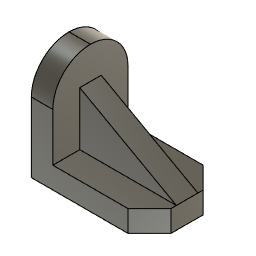
A1 (Autodesk Fusion 360 design; units mm, degrees)
Autodesk Fusion 360 part; units mm, degrees
note: some values were not read from the file. Set by a fixed rule: which sketch regions a step uses.
sketch "Sketch1" plane through (0, 0, 0) normal (0, 0, 1) x (1, 0, 0)
  line L0 (-20.0087, 11.2989) -> (639.9913, 11.2989)
  line L1 (639.9913, 11.2989) -> (639.9913, -408.7011)
  line L2 (639.9913, -408.7011) -> (-20.0087, -408.7011)
  line L3 (-20.0087, -408.7011) -> (-20.0087, 11.2989)
  line L4 (519.9913, -288.7011) -> (639.9913, -288.7011)
  line L5 (639.9913, -288.7011) -> (639.9913, -408.7011)
  line L6 (639.9913, -408.7011) -> (519.9913, -408.7011)
  line L7 (519.9913, -408.7011) -> (519.9913, -288.7011)
  line L8 (519.9913, 11.2989) -> (639.9913, 11.2989)
  line L9 (639.9913, 11.2989) -> (639.9913, -108.7011)
  line L10 (639.9913, -108.7011) -> (519.9913, -108.7011)
  line L11 (519.9913, -108.7011) -> (519.9913, 11.2989)
  line L12 (519.9913, -408.7011) -> (639.9913, -288.7011)
  line L13 (519.9913, 11.2989) -> (639.9913, -108.7011)
  dimension "d1" = 660
  dimension "d2" = 420
  dimension "d3" = 120
  dimension "d4" = 120
  dimension "d5" = 120
  dimension "d6" = 120
  constraint horizontal L0
  constraint vertical L1
  constraint horizontal L2
  constraint vertical L3
  constraint horizontal L4
  constraint vertical L5
  constraint horizontal L6
  constraint vertical L7
  constraint collinear L2 L6
  constraint collinear L1 L5
  constraint horizontal L8
  constraint vertical L9
  constraint horizontal L10
  constraint vertical L11
  constraint coincident L0 L8.start
  constraint collinear L1 L9
  measures "d1" distance of L0.start L0.end
  measures "d2" distance of L0.start L2.end
  measures "d3" distance of L4.start L4.end
  measures "d4" distance of L4.start L6.end
  measures "d5" distance of L8.start L0.end
  measures "d6" distance of L8.start L10.end
extrude "Extrude2" add sketch "Sketch1" along normal blind 120 contours L0 L1 L2 L3 L4 L7 L10 L11 | L10 L11 L13 | L4 L7 L12 makes body 1
sketch "Sketch2" plane through (0, 0, 120) normal (0, 0, 1) x (-1, 0, 0)
  line L0 (-519.9913, 408.7011) -> (-639.9913, 288.7011)
  line L1 (-639.9913, 288.7011) -> (-639.9913, 108.7011)
  line L2 (-639.9913, 108.7011) -> (-519.9913, -11.2989)
  line L3 (-519.9913, -11.2989) -> (20.0087, -11.2989)
  line L4 (20.0087, -11.2989) -> (20.0087, 408.7011)
  line L5 (20.0087, 408.7011) -> (-519.9913, 408.7011)
  line L6 (20.0087, -11.2989) -> (-99.9913, -11.2989)
  line L7 (-99.9913, -11.2989) -> (-99.9913, 408.7011)
  line L8 (-99.9913, 408.7011) -> (20.0087, 408.7011)
  line L9 (20.0087, 408.7011) -> (20.0087, -11.2989)
  dimension "d11" = 120
  constraint horizontal L6
  constraint vertical L7
  constraint horizontal L8
  constraint vertical L9
  constraint coincident L3.end L4.start
  measures "d11" distance of L3.end L6.end
extrude "Extrude3" add sketch "Sketch2" along normal blind 270 contours L3 L4 L5 L6 L7 L8 L9 bodies 1
sketch "Sketch3" plane through (0, -408.7011, 0) normal (0, -1, 0) x (1, 0, 0)
  line L0 (-20.0087, 0) -> (519.9913, 0)
  line L1 (519.9913, 0) -> (519.9913, 120)
  line L2 (519.9913, 120) -> (99.9913, 120)
  line L3 (99.9913, 120) -> (99.9913, 390)
  line L4 (99.9913, 390) -> (-20.0087, 390)
  line L5 (-20.0087, 390) -> (-20.0087, 0)
  line L6 (99.9913, 120) -> (99.9913, 420)
  line L7 (99.9913, 120) -> (639.9913, 120)
  line L8 (99.9913, 420) -> (639.9913, 120)
  dimension "d14" = 300
  dimension "d15" = 540
  constraint coincident L2.end L3.start
  constraint perpendicular L4 L6
  constraint perpendicular L1 L7
  measures "d14" distance of L2.end L6.end
  measures "d15" distance of L2.end L7.end
extrude "Extrude4" add sketch "Sketch3" along normal blind 120 separate body contours L2 L3 L6 L7 L8 makes body 2
move_body "Move1" bodies 2 to x (1, 0, 0) y (0, 1, 0) z (0, 0, 1) at (-487.7424, -224.6451, -38.3321)
move_body "Move2" bodies 2 to x (1, 0, 0) y (0, 1, 0) z (0, 0, 1) at (490, 500, 40)
move_body "Move3" bodies 2 to x (1, 0, 0) y (0, 1, 0) z (0, 0, 1) at (0, -5, 0)
sketch "Sketch5" plane through (-20.0087, 0, 0) normal (-1, 0, 0) x (0, -1, 0)
  line L0 (-11.2989, 0) -> (408.7011, 0)
  line L1 (408.7011, 0) -> (408.7011, 390)
  line L2 (408.7011, 390) -> (-11.2989, 390)
  line L3 (-11.2989, 390) -> (-11.2989, 0)
  line L4 (-11.2989, 390) -> (408.7011, 390)
  line L5 (408.7011, 390) -> (408.7011, 390.0002)
  line L6 (198.6557, 600.0002) -> (198.7011, 600.0002)
  line L7 (-11.2988, 390.0783) -> (-11.2989, 390)
  arc A0 (198.7011, 600.0002) -> (-11.2988, 390.0783) centre (198.7011, 390.0002) ccw
  arc A1 (408.7011, 390.0002) -> (198.6557, 600.0002) centre (198.7011, 390.0002) ccw
  point P0 (-11.2208, 600)
  dimension "d28" = 420
  dimension "d29" = 210
  dimension "d30" = 210
  dimension "d31" = 210
  constraint horizontal L4
  constraint vertical L5
  constraint coincident L2.end L3.start
  constraint coincident P0 L7
  constraint tangent L7 A0
  constraint tangent L5 A1
  constraint tangent L6 A1
  measures "d28" distance of L2.end L1.end
  measures "d29" distance of L2.end P0
  measures "d30" radius of A0
  measures "d31" radius of A1
extrude "Extrude5" add sketch "Sketch5" against normal blind 120 contours L2 L4 L6 L7 A0 A1 bodies 1
combine "Combine1" operation add target body 2 tool bodies 1 makes body 3 at (159.9913, -128.7011, 0)
move_body "Move4" bodies 2 to x (1, 0, 0) y (0, 1, 0) z (0, 0, 1) at (-2.5, 0, -1.6)
move_body "Move5" bodies 2 to x (1, 0, 0) y (0, 1, 0) z (0, 0, 1) at (0.4, 0, 0)
move_body "Align1" bodies 2 to x (1, 0, 0) y (0, 1, 0) z (0, 0, 1) at (-0.1576, 0, -0.0679)
combine "Combine5" operation add target body 2 tool bodies 3
named bodies: "A1"
